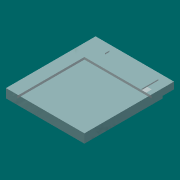
# Autodesk Inventor part: lens
Saved by Autodesk Inventor 2016 (Build 200138000, 138)
## iProperties
Created: 2016-02-09
Part Number: lens
Material: Glass
Document SubType Name: Modeling
Designer: Sawaiz
Density: 2.18 g/cm^3
Appearance: Clear
Author: Sawaiz
Autodesk Inventor part; units mm, degrees
sketch "Sketch1" plane through (0, 0, 0) normal (0, 0, 1) x (1, 0, 0)
  line L0 (-1.5, 1.5) -> (1.5, 1.5) projected
  line L1 (1.5, 1.5) -> (1.5, -1.5) projected
  line L2 (1.5, -1.5) -> (-1.5, -1.5) projected
  line L3 (-1.5, -1.5) -> (-1.5, 1.5) projected
  line L4 (-1.75, -1.75) -> (-1.75, 1.75) projected
  line L5 (1.75, -1.75) -> (-1.75, -1.75) projected
  line L6 (1.75, 1.75) -> (1.75, -1.75) projected
  line L7 (-1.75, 1.75) -> (1.75, 1.75) projected
  point P0 (0, 0)
ref_plane "Work Plane1" through (-2.25, -1.75, 0.1) normal (0, 0, 1) x (1, 0, 0)
extrude "Extrusion1" add sketch "Sketch1" along normal up to surface (0.1 mm away)
sketch "Sketch2" plane through (-1.75, 1.75, 0.1) normal (0, 0, 1) x (1, 0, 0)
  line L0 (-0.5, -0.4937) -> (0, -0.4937) projected
  line L1 (0, 0) -> (0, -0.4937) projected
  line L2 (-0.5, 0) -> (0, 0) projected
  line L3 (-0.5, -0.4937) -> (-0.5, 0) projected
  line L4 (-0.5, -2.3875) -> (-0.3, -2.3875) projected
  line L5 (-0.3, -2.3875) -> (-0.3, -2.8875) projected
  line L6 (-0.3, -2.8875) -> (-0.5, -2.8875) projected
  line L7 (-0.5, -3.5) -> (-0.5, -2.8875) projected
  line L8 (0, -3.5) -> (-0.5, -3.5) projected
  line L9 (0, -0.6937) -> (0, -3.5) projected
  line L10 (0, -0.6937) -> (-0.5, -0.6937) projected
  line L11 (-0.5, -2.3875) -> (-0.5, -0.6937) projected
  line L12 (0.25, -0.25) -> (0.25, -0.4937) projected
  line L13 (0.25, -0.4937) -> (0.25, -0.6937) projected
  line L14 (0.25, -0.6937) -> (0.25, -3.25) projected
  line L15 (0.25, -3.25) -> (3.25, -3.25) projected
  line L16 (3.25, -3.25) -> (3.25, -0.25) projected
  line L17 (3.25, -0.25) -> (0.25, -0.25) projected
  point P0 (1.75, -1.75)
ref_plane "Work Plane2" through (-2.25, 1.0563, 0.15) normal (0, 0, 1) x (1, 0, 0)
extrude "Extrusion2" add sketch "Sketch2" along normal up to surface (0.05 mm away)
sketch "Sketch3" plane through (1.75, -1.75, 0.1) normal (0, 0, 1) x (1, 0, 0)
  line L0 (-4, 2.8063) -> (-4, 3.0063) projected
  line L1 (-4, 2.8063) -> (-3.25, 2.8063) projected
  line L2 (-3.25, 2.8063) -> (-3.25, 3.0063) projected
  line L3 (-3.25, 3.0063) -> (-4, 3.0063) projected
  line L4 (-0.25, 0.25) -> (-0.25, 3.25) projected
  line L5 (-3.25, 0.25) -> (-0.25, 0.25) projected
  line L6 (-3.25, 3.25) -> (-3.25, 0.25) projected
  line L7 (-0.25, 3.25) -> (-3.25, 3.25) projected
  line L8 (-3.5, 3.5) -> (0, 3.5) projected
  line L9 (-3.5, 3.0063) -> (-3.5, 3.5) projected
  line L10 (-3.5, 2.8063) -> (-3.5, 3.0063) projected
  line L11 (-3.5, 0) -> (-3.5, 2.8063) projected
  line L12 (0, 0) -> (-3.5, 0) projected
  line L13 (0, 3.5) -> (0, 0) projected
  line L14 (-3.5, 3.0063) -> (-3.25, 3.0063)
  line L15 (-3.5, 2.8063) -> (-3.25, 2.8063)
  point P0 (-1.75, 1.75)
  constraints: 4 end point, 2 collinear
extrude "Extrusion3" add sketch "Sketch3" along normal up to surface (0.05 mm away) contours L1 L6 L5 L4 L7 L3 L9 L8 L13 L12 L11
sketch "Sketch4" plane through (-2.25, -1.75, 0.15) normal (0, 0, 1) x (1, 0, 0)
  line L0 (0, 1.1125) -> (0, 2.8063) projected
  line L1 (0.2, 1.1125) -> (0, 1.1125) projected
  line L2 (0.2, 0.6125) -> (0.2, 1.1125) projected
  line L3 (0, 0.6125) -> (0.2, 0.6125) projected
  line L4 (0, 0) -> (0, 0.6125) projected
  line L5 (4, 0) -> (0, 0) projected
  line L6 (4, 3.5) -> (4, 0) projected
  line L7 (0, 3.5) -> (4, 3.5) projected
  line L8 (0, 3.0063) -> (0, 3.5) projected
  line L9 (0.75, 3.0063) -> (0, 3.0063) projected
  line L10 (0.75, 2.8063) -> (0.75, 3.0063) projected
  line L11 (0, 2.8063) -> (0.75, 2.8063) projected
  line L12 (0, 2.8063) -> (0, 3.0063) projected
  line L13 (0, 2.8063) -> (0.75, 2.8063) projected
  line L14 (0.75, 2.8063) -> (0.75, 3.0063) projected
  line L15 (0.75, 3.0063) -> (0, 3.0063) projected
  line L16 (0, 0.6125) -> (0, 1.1125) projected
  line L17 (0, 0.6125) -> (0.2, 0.6125) projected
  line L18 (0.2, 0.6125) -> (0.2, 1.1125) projected
  line L19 (0.2, 1.1125) -> (0, 1.1125) projected
  point P0 (2.25, 1.75)
ref_plane "Work Plane3" through (-2.425, -1.925, 0.4) normal (0, 0, 1) x (1, 0, 0)
extrude "Extrusion4" add sketch "Sketch4" along normal up to surface (0.25 mm away)
body "Solid1"
